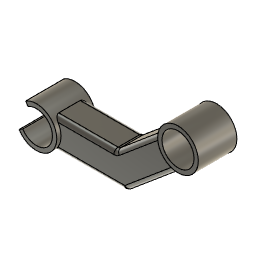
Arm v1 (Autodesk Fusion 360 design; units mm, degrees)
Autodesk Fusion 360 part; units mm, degrees
note: some values were not read from the file. Set by a fixed rule: which sketch regions a step uses.
sketch "Sketch1" plane through (0, 0, 0) normal (0, 1, 0) x (1, 0, 0)
  line L0 (0, 0) -> (40, 0)
  line L1 (34.9044, -14) -> (0, -14)
  line L2 (0, -14) -> (0, 0)
  line L3 (61.6428, -36.4361) -> (34.9044, -14)
  line L4 (70.6418, -25.7115) -> (61.6428, -36.4361)
  line L5 (40, 0) -> (70.6418, -25.7115)
  dimension "d1" = 40
  dimension "d2" = 14
  dimension "d3" = 14
  dimension "d4" = 40
  dimension "d5" = 140
  constraint horizontal L0
  constraint horizontal L1
  constraint vertical L2
  constraint coincident L0.start L2.end
  constraint parallel L3 L5
  constraint perpendicular L3 L4
  measures "d1" distance of L0.start L0.end
  measures "d2" distance of L0.start L1.end
  measures "d3" distance of L3.start L4.start
  measures "d4" distance of L0.end L4.start
  measures "d5" angle of L1 L3
extrude "Extrude1" add sketch "Sketch1" along normal blind 14
fillet "Fillet1" radius 2 10 edges at (17.4522, 0, 14) (20, 0, 0) (34.9044, 7, 14) (48.2736, 0, 25.2181) (17.4522, 14, 14) (55.3209, 0, 12.8558) (48.2736, 14, 25.2181) (55.3209, 14, 12.8558) (20, 14, 0) (40, 7, 0)
shell "Shell1" thickness 1 removed faces 2 at (0, 5.3333, 9.3333) at (66.7851, 5.3333, 30.3078)
sketch "Sketch2" plane through (0, 0, 0) normal (0, -1, 0) x (1, 0, 0)
  line L0 (39.2721, 2) -> (69.3562, 27.2436)
  line L1 (69.3562, 27.2436) -> (62.9283, 34.904)
  line L2 (62.9283, 34.904) -> (36.7476, 12.9358)
  arc A0 (34.1765, 12) -> (36.7476, 12.9358) centre (34.1765, 16) ccw
  line L3 (34.1765, 12) -> (0, 12)
  line L4 (0, 12) -> (0, 2)
  line L5 (0, 2) -> (39.2721, 2)
  circle A1 centre (0, 7) radius 9.5
  circle A2 centre (66.1423, 31.0738) radius 9.5
  dimension "d11" = 19
  dimension "d12" = 19
  constraint midpoint L4 A1.centre
  constraint midpoint L1 A2.centre
  measures "d11" diameter of A1
  measures "d12" diameter of A2
extrude "Extrude2" add sketch "Sketch2" along normal blind -16 and the other way blind -2 contours L0 L1 L2 A2 | L0 L1 L2 A2 | L3 L4 L5 A1 | L3 L4 L5 A1
sketch "Sketch3" plane through (0, -2, 0) normal (0, -1, 0) x (1, 0, 0)
  circle A0 centre (66.1423, 31.0738) radius 9.5
  circle A1 centre (66.1423, 31.0738) radius 7.5
  dimension "d17" = -2
extrude "Extrude3" cut sketch "Sketch3" against normal through all contours A1
sketch "Sketch4" plane through (0, -2, 0) normal (0, -1, 0) x (1, 0, 0)
  circle A0 centre (0, 7) radius 9.5
  line L0 (0, 7) -> (-5, 15.0777)
  circle A1 centre (0, 7) radius 7.5
  line L1 (0, 7) -> (-8.0777, 2)
  line L2 (0, 7) -> (0, 10.0999)
  line L3 (0, 10.0999) -> (0, 16.5)
  dimension "d19" = -2
  dimension "d20" = 90
  dimension "d21" = 5
  constraint coincident A0.centre L0.start
  constraint coincident A0 L0.end
  constraint coincident A0 L1.end
  constraint vertical L2
  constraint coincident A0 L3.end
  constraint parallel L2 L3
  measures "d20" angle of L0 L1
  measures "d21" horizontal distance of L0.end L3.end
extrude "Extrude4" cut sketch "Sketch4" against normal blind 40 contours A0 L0 A1 L1 | L0 A1 L2 L3 | A1 L1 L2 L3 | L0 A1 L1
